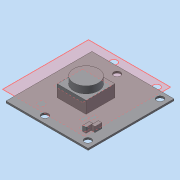
# Autodesk Inventor part: Board
Saved by Autodesk Inventor 2016 SP1 (Build 200210100, 210)
## iProperties
Created: 2016-03-20
Part Number: Board
Material: Generic
Document SubType Name: Modeling
Designer: Mohamed A.
Density: 1 g/cm^3
Appearance: Default
Author: Mohamed A.
Autodesk Inventor part; units mm, degrees
ref_plane "YZ Plane" through (0, 0, 0) normal (1, 0, 0) x (0, 1, 0)
ref_plane "XZ Plane" through (0, 0, 0) normal (0, 1, 0) x (-1, 0, 0)
ref_plane "XY Plane" through (0, 0, 0) normal (0, 0, 1) x (1, 0, 0)
sketch "Sketch1" plane through (0, 0, 0) normal (0, 0, 1) x (1, 0, 0)
  line L0 (-11.95, 12.5) -> (11.95, 12.5)
  line L1 (11.95, 12.5) -> (11.95, -12.5)
  line L2 (11.95, -12.5) -> (-11.95, -12.5)
  line L3 (-11.95, -12.5) -> (-11.95, 12.5)
  line L4 (-11.95, 12.5) -> (11.95, -12.5) construction
  line L5 (11.95, 12.5) -> (-11.95, -12.5) construction
  circle A0 centre (9.9, -10.5) radius 1
  circle A1 centre (-2.6, -10.5) radius 1
  line L6 (11.5332, -10.5) -> (-16.0268, -10.5) construction
  line L7 (9.9, -13.3661) -> (9.9, 11.2852) construction
  line L8 (11.2708, 10.5) -> (-4.8598, 10.5) construction
  circle A2 centre (9.9, 10.5) radius 1
  line L9 (-2.6, -15.3332) -> (-2.6, 11.9823) construction
  circle A3 centre (-2.6, 10.5) radius 1
  point P0 (0, 0)
  dimension "d0" = 23.9
  dimension "d1" = 25
  dimension "d2" = 2
  dimension "d3" = 21.85
  dimension "d5" = 2
  dimension "d6" = 9.35
  dimension "d7" = 2
  dimension "d8" = 23
  dimension "d9" = 2
  dimension "d10" = 2
  constraints: 20 end point, 8 point on line, 4 centre point, 3 horizontal, 2 midpoint, 2 parallel, 2 perpendicular, 1 vertical
  measures "d0" distance of L1.end L2.end
  measures "d1" distance of L0.end L1.end
  measures "d2" diameter of A0
  measures "d3" distance from line of L3 A0.centre
  measures "d5" diameter of A1
  measures "d6" distance from line of L3 A1.centre
  measures "d7" distance between parallel lines of L2 L6
  measures "d8" distance between parallel lines of L2 L8
  measures "d9" diameter of A2
  measures "d10" diameter of A3
extrude "Extrusion1" add sketch "Sketch1" along normal blind 0.5
sketch "Sketch2" plane through (0, 0, 0.5) normal (0, 0, 1) x (1, 0, 0)
  line L0 (-16.73, 0) -> (16.73, 0) construction
  line L1 (-5.35, 4.2) -> (3.05, 4.2)
  line L2 (3.05, 4.2) -> (3.05, -4.2)
  line L3 (3.05, -4.2) -> (-5.35, -4.2)
  line L4 (-5.35, -4.2) -> (-5.35, 4.2)
  line L5 (-5.35, 4.2) -> (3.05, -4.2) construction
  line L6 (3.05, 4.2) -> (-5.35, -4.2) construction
  line L7 (-11.95, 12.5) -> (-11.95, -12.5) projected
  point P0 (0, 0)
  point P1 (-1.15, 0)
  dimension "d13" = 8.4
  dimension "d14" = 8.4
  dimension "d15" = 6.6
  constraints: 12 end point, 2 midpoint, 2 parallel, 1 horizontal, 1 perpendicular, 1 point on line
  measures "d13" distance of L2.end L3.end
  measures "d14" distance of L1.end L2.end
  measures "d15" distance between parallel lines of L7 L4
extrude "Extrusion2" add sketch "Sketch2" along normal blind 3.5
sketch "Sketch3" plane through (0, 0, 4) normal (0, 0, 1) x (1, 0, 0)
  line L0 (-5.35, 4.2) -> (3.05, 4.2) construction
  line L1 (-5.35, 4.2) -> (3.05, -4.2) construction
  line L2 (-5.35, -4.2) -> (3.05, -4.2) construction
  line L3 (3.05, 4.2) -> (-5.35, -4.2) construction
  circle A0 centre (-1.15, 0) radius 3.6
  point P0 (0, 0)
  dimension "d18" = 7.2
  constraints: 4 end point, 1 centre point, 1 midpoint
  measures "d18" diameter of A0
extrude "Extrusion3" add sketch "Sketch3" along normal blind 2
sketch "Sketch4" plane through (0, 0, 0.5) normal (0, 0, 1) x (1, 0, 0)
  line L0 (6.85, -7) -> (7.85, -7)
  line L1 (7.85, -7) -> (7.85, -9)
  line L2 (7.85, -9) -> (6.85, -9)
  line L3 (6.85, -9) -> (6.85, -7)
  line L4 (7.95, -5.5) -> (8.95, -5.5)
  line L5 (8.95, -5.5) -> (8.95, -7.5)
  line L6 (8.95, -7.5) -> (7.95, -7.5)
  line L7 (7.95, -7.5) -> (7.95, -5.5)
  line L8 (-11.95, -12.5) -> (11.95, -12.5) projected
  line L9 (11.95, -12.5) -> (11.95, 12.5) projected
  point P0 (0, 0)
  dimension "d21" = 3.5
  dimension "d22" = 1
  dimension "d23" = 2
  dimension "d25" = 3
  dimension "d26" = 1
  dimension "d27" = 2
  dimension "d28" = 5
  dimension "d31" = 0.1
  constraints: 16 end point, 4 parallel, 2 horizontal, 2 perpendicular
  measures "d21" distance between parallel lines of L8 L2
  measures "d22" distance between parallel lines of L3 L1
  measures "d23" distance between parallel lines of L2 L0
  measures "d25" distance between parallel lines of L9 L5
  measures "d26" distance between parallel lines of L7 L5
  measures "d27" distance between parallel lines of L6 L4
  measures "d28" distance between parallel lines of L8 L6
  measures "d31" distance between parallel lines of L7 L1
extrude "Extrusion4" add sketch "Sketch4" along normal blind 1.5
body "Solid1"
